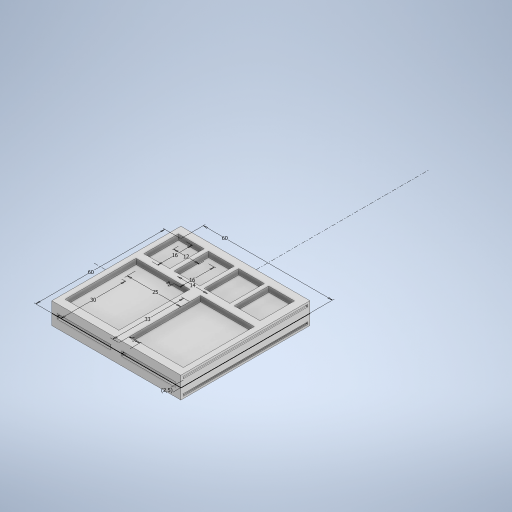
# Autodesk Inventor part: cotieni SD-micro SD
Saved by Autodesk Inventor 2023 (Build 270158000, 158)
## iProperties
Created: 2023-07-25
Part Number: cotieni SD-micro SD
Material: Generico
Document SubType Name: Modeling
Designer: Admin
Density: 1 g/cm^3
Appearance: Default
Author: Admin
Autodesk Inventor part; units mm, degrees
ref_plane "YZ Plane" through (0, 0, 0) normal (1, 0, 0) x (0, 1, 0)
ref_plane "XZ Plane" through (0, 0, 0) normal (0, 1, 0) x (-1, 0, 0)
ref_plane "XY Plane" through (0, 0, 0) normal (0, 0, 1) x (1, 0, 0)
sketch "Schizzo1" plane through (0, 0, 0) normal (0, 1, 0) x (-1, 0, 0)
  line L0 (30, 30) -> (-30, 30)
  line L1 (-30, 30) -> (-30, -30)
  line L2 (-30, -30) -> (30, -30)
  line L3 (30, -30) -> (30, 30)
  line L4 (0, 0) -> (0, -115.6454) construction
  line L5 (0, 0) -> (41.0796, 0) construction
  line L6 (27.5, 26.3333) -> (2.5, 26.3333)
  line L7 (2.5, 26.3333) -> (2.5, -6.6667)
  line L8 (2.5, -6.6667) -> (27.5, -6.6667)
  line L9 (27.5, -6.6667) -> (27.5, 26.3333)
  line L10 (30, 30) -> (30, 26.3333) construction
  line L11 (30, 26.3333) -> (27.5, 26.3333) construction
  line L12 (15.5, -10.3333) -> (15.5, -26.3333)
  line L13 (15.5, -26.3333) -> (27.5, -26.3333)
  line L14 (27.5, -26.3333) -> (27.5, -10.3333)
  line L15 (27.5, -10.3333) -> (15.5, -10.3333)
  line L16 (27.5, -6.6667) -> (27.5, -10.3333) construction
  line L17 (27.5, -10.3333) -> (30, -10.3333) construction
  line L18 (1.5, -10.3333) -> (1.5, -26.3333)
  line L19 (1.5, -26.3333) -> (13.5, -26.3333)
  line L20 (13.5, -10.3333) -> (1.5, -10.3333)
  line L21 (15.5, -10.3333) -> (13.5, -10.3333) construction
  line L22 (-2.5, -6.6667) -> (-27.5, -6.6667)
  line L23 (-27.5, -6.6667) -> (-27.5, 26.3333)
  line L24 (-27.5, 26.3333) -> (-2.5, 26.3333)
  line L25 (-2.5, 26.3333) -> (-2.5, -6.6667)
  line L26 (-14.5, -10.3333) -> (-14.5, -26.3333)
  line L27 (-14.5, -26.3333) -> (-26.5, -26.3333)
  line L28 (-26.5, -26.3333) -> (-26.5, -10.3333)
  line L29 (-26.5, -10.3333) -> (-14.5, -10.3333)
  line L30 (-0.5, -10.3333) -> (-0.5, -26.3333)
  line L31 (-12.5, -26.3333) -> (-12.5, -10.3333)
  line L32 (-12.5, -10.3333) -> (-0.5, -10.3333)
  line L33 (-0.5, -26.3333) -> (-12.5, -26.3333)
  line L34 (4.1, -0.1) -> (3.9, -0.1) construction
  line L35 (1.5, -10.3333) -> (-0.5, -10.3333) construction
  line L36 (-12.5, -10.3333) -> (-14.5, -10.3333) construction
  line L37 (2.5, 26.3333) -> (-2.5, 26.3333) construction
  line L38 (27.5, 30) -> (27.5, 0)
  line L39 (27.5, 0) -> (2.5, 0)
  line L40 (2.5, 0) -> (2.5, 30)
  line L41 (-27.5, 0) -> (-2.5, 0)
  line L42 (-2.5, 30) -> (-2.5, 0)
  line L43 (-2.5, 0) -> (-27.5, 0)
  line L44 (-27.5, 0) -> (-27.5, 30)
  line L45 (28.75, 30) -> (28.75, 26.3333) construction
  line L46 (27.5, -30) -> (27.5, -14)
  line L47 (27.5, -14) -> (15.5, -14)
  line L48 (15.5, -14) -> (15.5, -30)
  line L49 (27.5, -30) -> (27.5, -26.3333) construction
  line L50 (27.5, -26.3333) -> (30, -26.3333) construction
  line L51 (28.75, -26.3333) -> (28.75, -30) construction
  line L52 (15.5, -26.3333) -> (13.5, -26.3333) construction
  line L53 (-27.5, 26.3333) -> (-30, 26.3333) construction
  line L54 (13.5, -26.3333) -> (13.5, -10.3333)
  line L55 (1.5, -14) -> (1.5, -30)
  line L56 (13.5, -14) -> (1.5, -14)
  line L57 (13.5, -30) -> (13.5, -14)
  line L58 (-12.5, -14) -> (-12.5, -30)
  line L59 (-0.5, -14) -> (-12.5, -14)
  line L60 (-0.5, -30) -> (-0.5, -14)
  line L61 (-26.5, -14) -> (-26.5, -30)
  line L62 (-14.5, -14) -> (-26.5, -14)
  line L63 (-14.5, -30) -> (-14.5, -14)
  point P0 (0.4384, -30)
  point P1 (-4.1232, -30)
  point P2 (-2.5, 0)
  dimension "d2" = 25
  dimension "d3" = 33
  dimension "d6" = 12
  dimension "d26" = 60
  dimension "d46" = 30
  dimension "d47" = 16
  dimension "d61" = 60
  dimension "d62" = 2
  dimension "d63" = 16
  dimension "d66" = 14
  dimension "d71" = 5
  dimension "d82" = 2.5
  constraints: 130 end point, 22 perpendicular, 21 point on line, 16 parallel, 15 equal length, 7 horizontal, 4 collinear, 2 midpoint, 2 symmetric about line, 2 vertical, 23 other
  measures "d2" distance of L8.end L7.end
  measures "d3" distance of L7.end L6.end
  measures "d6" distance of L13.end L12.end
  measures "d26" distance of L2.end L0.start
  measures "d46" distance of L38.start L38.end
  measures "d47" distance of L46.start L46.end
  measures "d61" distance of L1.end L2.end
  measures "d62" distance of L12.start L20.start
  measures "d63" distance of L19.end L54.end
  measures "d66" distance of L47.end L55.start
  measures "d71" distance of L6.end L25.start
  measures "d82" distance of L24.start L53.end
extrude "Estrusione1" add sketch "Schizzo1" along normal mid plane 10 contours L3 L2 L46 L14 L15 L12 L48 L57 L54 L20 L18 L55 L60 L30 L32 L31 L58 L63 L26 L29 L28 L61 L1 L0 L44 L23 L22 L25 L42 L40 L7 L8 L9 L38 | L38 L6 L40 L0 | L2 L48 L13 L46 | L42 L24 L44 L0 | L2 L55 L19 L57 | L19 L18 L56 L54 | L2 L58 L33 L60 | L56 L18 L20 L54 | L61 L27 L63 L2
extrude "Estrusione2" add sketch "Schizzo1" along normal mid plane 5 contours L9 L39 L7 L6 | L9 L8 L7 L39 | L13 L12 L47 L14 | L25 L41 L23 L24 | L47 L12 L15 L14 | L25 L22 L23 L41 | L33 L31 L59 L30 | L28 L62 L26 L27 | L59 L31 L32 L30 | L28 L29 L26 L62
extrude "Estrusione10" cut sketch "Schizzo1" along normal mid plane 10 contours L19 L18 L56 L54 | L56 L18 L20 L54
extrude "Estrusione11" add sketch "Schizzo1" along normal mid plane 5 contours L19 L18 L56 L54 | L56 L18 L20 L54
extrude "Estrusione12" cut sketch "Schizzo1" along normal mid plane 1.2 contours L2 L48 L13 L46 | L13 L12 L47 L14 | L2 L55 L19 L57 | L19 L18 L56 L54 | L2 L58 L33 L60 | L61 L27 L63 L2 | L33 L31 L59 L30 | L28 L62 L26 L27
extrude "Estrusione13" cut sketch "Schizzo1" along normal mid plane 2.2 contours L38 L6 L40 L0 | L9 L39 L7 L6 | L42 L24 L44 L0 | L25 L41 L23 L24
sketch "Schizzo5" plane through (-30, -5, 30) normal (-1, 0, 0) x (0, 0, 1)
  line L0 (-60, 0) -> (-60, 10) projected
  line L1 (0, 0) -> (-60, 0) projected
  line L2 (-60, 10) -> (0, 10) projected
  line L3 (0, 0) -> (0, 10) projected
  line L4 (-60, 0) -> (-60, 10) construction
  line L5 (-60, 5) -> (-60, 1) construction
  line L6 (-60, 1) -> (-59, 1) construction
  line L7 (-59, 1) -> (-59, 2)
  line L8 (-59, 1) -> (-1, 1)
  line L9 (-1, 1) -> (-1, 2)
  line L10 (-1, 2) -> (-59, 2)
  line L11 (-30, 5) -> (-145.6454, 5) construction
  line L12 (-59, 9) -> (-59, 8)
  line L13 (-59, 9) -> (-1, 9)
  line L14 (-1, 9) -> (-1, 8)
  line L15 (-1, 8) -> (-59, 8)
  line L16 (-59.2, 2.2) -> (-59.2, 0.8)
  line L17 (-59.2, 0.8) -> (-0.8, 0.8)
  line L18 (-0.8, 0.8) -> (-0.8, 2.2)
  line L19 (-0.8, 2.2) -> (-59.2, 2.2)
  line L20 (-0.8, 9.2) -> (-59.2, 9.2)
  line L21 (-59.2, 9.2) -> (-59.2, 7.8)
  line L22 (-59.2, 7.8) -> (-0.8, 7.8)
  line L23 (-0.8, 7.8) -> (-0.8, 9.2)
  dimension "d83" = 10
  dimension "d84" = 4
  dimension "d85" = 1
  dimension "d86" = 1
  dimension "d87" = 60
  dimension "d88" = 58
  dimension "d89" = 1
  dimension "d90" = 0.2
  dimension "d91" = 0.2
  dimension "d108" = 1.4
  constraints: 36 end point, 4 symmetric about line, 3 perpendicular, 1 midpoint, 1 point on line, 1 vertical, 6 other
  measures "d83" distance of L0.start L0.end
  measures "d84" distance of L5.start L5.end
  measures "d85" distance of L5.end L6.end
  measures "d86" distance of L6.end L7.end
  measures "d87" distance of L1.start L0.start
  measures "d88" distance of L6.end L8.end
  measures "d89" distance of L8.end L9.end
  measures "d90" distance between parallel lines of L10 L19
  measures "d91" distance between parallel lines of L13 L20
  measures "d108" distance of L16.start L16.end
extrude "Estrusione14" cut sketch "Schizzo5" against normal blind 1.5 contours L7 L10 L9 L8 | L13 L14 L15 L12 | L19 L18 L17 L16 | L23 L22 L21 L20
extrude "Estrusione15" add sketch "Schizzo5" against normal blind 0.5 contours L19 L18 L17 L16 | L23 L22 L21 L20
sketch "Schizzo8" plane through (30, -5, -30) normal (1, 0, 0) x (0, 0, -1)
  line L0 (-60, 3.9) -> (-60, 6.1) construction
  line L1 (-60, 5) -> (-60, 1) construction
  line L2 (-1, 1) -> (-59, 1) construction
  line L3 (-60, 1) -> (-59, 1) construction
  line L4 (-59, 1) -> (-59, 2) projected
  line L5 (-59, 1) -> (-59, 2)
  line L6 (0, 0) -> (0, 10) projected
  line L7 (-1, 2) -> (-1, 1) projected
  line L8 (-59, 2) -> (-1, 2) projected
  line L9 (-1, 1) -> (-1, 2)
  line L10 (-1, 1) -> (-59, 1)
  line L11 (-59.2, 0.8) -> (-59.2, 2.2) projected
  line L12 (-59, 2) -> (-1, 2)
  line L13 (-59.2, 2.2) -> (-59.2, 0.8)
  line L14 (-59.2, 0.8) -> (-0.8, 0.8)
  line L15 (-0.8, 0.8) -> (-0.8, 2.2)
  line L16 (-0.8, 2.2) -> (-59.2, 2.2)
  line L17 (-60, 5) -> (0, 5) projected
  line L18 (-59, 9) -> (-59, 8)
  line L19 (-59, 9) -> (-59, 8)
  line L20 (-1, 8) -> (-1, 9)
  line L21 (-1, 9) -> (-1, 8)
  line L22 (-1, 9) -> (-59, 9)
  line L23 (-59.2, 9.2) -> (-59.2, 7.8)
  line L24 (-59, 8) -> (-1, 8)
  line L25 (-59.2, 7.8) -> (-59.2, 9.2)
  line L26 (-59.2, 9.2) -> (-0.8, 9.2)
  line L27 (-0.8, 9.2) -> (-0.8, 7.8)
  line L28 (-0.8, 7.8) -> (-59.2, 7.8)
  point P0 (-30, 5)
  dimension "d101" = 4
  dimension "d102" = 1
  dimension "d103" = 0.2
  constraints: 42 end point, 10 symmetric about line, 2 collinear, 2 perpendicular, 1 midpoint, 1 vertical, 3 other
  measures "d101" distance of L1.start L1.end
  measures "d102" distance of L1.end L2.end
  measures "d103" distance between parallel lines of L4 L13
extrude "Estrusione16" cut sketch "Schizzo8" against normal blind 1.5 contours L4 L8 L7 L10 | L11 L16 L15 L14 | L22 L20 L24 L18 | L26 L27 L28 L23
extrude "Estrusione17" add sketch "Schizzo8" against normal blind 0.5
